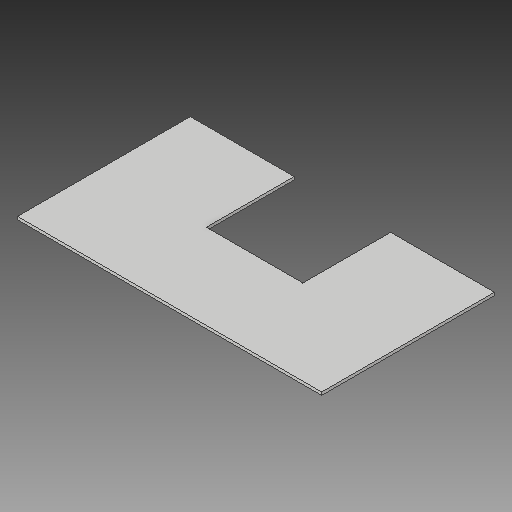
# Autodesk Inventor part: Electronics Board
Saved by Autodesk Inventor 2018.2 (Build 222227000, 227)
## iProperties
Created: 2018-01-29
Part Number: Electronics Board
Material: Generic
Document SubType Name: Modeling
Designer: Orangeracer
Density: 1 g/cm^3
Appearance: Default
Mass: 1319.97 g
Surface Area: 4313.09 cm^2
Volume: 1319.97 cm^3
Author: Orangeracer
Autodesk Inventor part; units mm, degrees
ref_plane "YZ Plane" through (0, 0, 0) normal (1, 0, 0) x (0, 1, 0)
ref_plane "XZ Plane" through (0, 0, 0) normal (0, 1, 0) x (-1, 0, 0)
ref_plane "XY Plane" through (0, 0, 0) normal (0, 0, 1) x (1, 0, 0)
sketch "Sketch1" plane through (0, 0, 0) normal (0, 1, 0) x (-1, 0, 0)
  line L0 (0, 0) -> (-660.4, 0)
  line L1 (-660.4, 0) -> (-660.4, 375.2088)
  line L2 (-660.4, 375.2088) -> (0, 375.2088)
  line L3 (0, 375.2088) -> (0, 0)
  dimension "d0" = 660.4
  dimension "d1" = 375.2088
  constraints: 8 end point, 2 parallel, 1 horizontal, 1 perpendicular
  measures "d0" distance of L1.end L2.end
  measures "d1" distance of L0.end L1.end
extrude "Extrusion1" add sketch "Sketch1" along normal blind 6.35
sketch "Sketch2" plane through (0, 0, 0) normal (0, -1, 0) x (1, 0, 0)
  line L0 (660.4, 0) -> (0, 0) projected
  line L1 (225.425, 0) -> (434.975, 0)
  line L2 (434.975, 0) -> (434.975, 190.5)
  line L3 (434.975, 190.5) -> (225.425, 190.5)
  line L4 (225.425, 190.5) -> (225.425, 0)
  line L5 (0, 375.2088) -> (0, 0) projected
  line L6 (660.4, 0) -> (660.4, 375.2088) projected
  dimension "d4" = 209.55
  dimension "d5" = 190.5
  dimension "d6" = 225.425
  dimension "d7" = 225.425
  constraints: 8 end point, 2 parallel, 1 horizontal, 1 perpendicular, 1 point on line
  measures "d4" distance of L2.end L3.end
  measures "d5" distance of L1.end L2.end
  measures "d6" distance between parallel lines of L5 L4
  measures "d7" distance between parallel lines of L6 L2
extrude "Extrusion2" cut sketch "Sketch2" against normal blind 6.35
body "Solid1"
